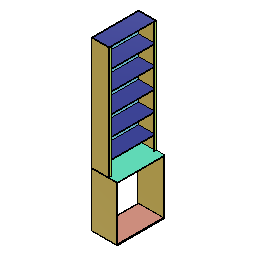
MS_BookShelves (Autodesk Fusion 360 design; units mm, degrees)
Autodesk Fusion 360 part; units mm, degrees
sketch "Part List" plane through (0, 0, 0) normal (1, 0, 0) x (0, 1, 0)
  line L0 (-117.4604, 5.2821) -> (-27.4764, 5.2821) construction
  line L1 (-27.4764, 5.2821) -> (-27.4764, 106.5384) construction
  line L2 (-27.4764, 106.5384) -> (-117.4604, 106.5384) construction
  line L3 (-117.4604, 106.5384) -> (-117.4604, 5.2821) construction
  dimension "d1" = 2
sketch "Room" plane through (0, 0, 0) normal (0, 0, 1) x (1, 0, 0)
  line L0 (922.3375, 3178.175) -> (2225.675, 3178.175) construction
  line L1 (0, 3178.175) -> (922.3375, 3178.175) construction
  line L2 (2225.675, 3178.175) -> (3114.675, 3178.175) construction
  line L3 (2259.0125, 0) -> (1363.6625, 0) construction
  line L4 (1363.6625, 46.449) -> (2259.0125, 46.449) construction
  line L5 (3114.675, 3178.175) -> (3630.6125, 3178.175) construction
  line L6 (0, 0) -> (0, 3178.175) construction
  line L7 (1363.6625, 0) -> (1363.6625, 46.449) construction
  line L8 (58.5758, 2317.75) -> (0, 2317.75) construction
  line L9 (0, 2403.475) -> (58.5758, 2403.475) construction
  line L10 (58.5758, 2403.475) -> (58.5758, 2317.75) construction
  line L11 (140.5097, 3178.175) -> (140.5097, 2420.9375) construction
  line L12 (0, 2317.75) -> (0, 2403.475) construction
  line L13 (0, 0) -> (3648.075, 0) construction
  line L14 (2259.0125, 46.449) -> (2259.0125, 0) construction
  point P0 (0, 2403.475)
  point P1 (0, 2317.75)
  point P2 (2259.0125, 0)
  point P3 (1363.6625, 0)
  dimension "d2" = 3648.075
  dimension "d3" = 895.35
  dimension "d4" = 1363.6625
  dimension "d5" = 1389.0625
  dimension "d6" = 3178.175
  dimension "d7" = 922.3375
  dimension "d8" = 1303.3375
  dimension "d9" = 889
  dimension "d10" = 515.9375
  dimension "d11" = 3630.6125
  dimension "d12" = 774.7
  dimension "d13" = 85.725
  dimension "d14" = 757.2375
  dimension "d15" = 90
  constraint coincident L6.start L13.start
  constraint horizontal L13
  constraint coincident P3 L13
  constraint coincident P2 L13
  constraint horizontal L3
  constraint vertical L7
  constraint horizontal L4
  constraint vertical L14
  constraint coincident P2 L3.start
  constraint perpendicular L6 L13
  constraint perpendicular L1 L6
  constraint parallel L0 L1
  constraint parallel L0 L2
  constraint parallel L2 L5
  constraint coincident P0 L6
  constraint coincident P1 L6
  constraint horizontal L9
  constraint vertical L10
  constraint horizontal L8
  constraint vertical L12
  constraint coincident P0 L9.start
  constraint coincident L11.start L1
  constraint perpendicular L1 L11
  measures "d2" distance of L13.end L6.start
  measures "d3" distance of P2 P3
  measures "d4" distance of L6.start P3
  measures "d5" distance of L13.end P2
  measures "d6" distance of L6.start L1.start
  measures "d7" distance of L1.start L0.start
  measures "d8" distance of L0.start L0.end
  measures "d9" distance of L0.end L2.end
  measures "d10" distance of L2.end L5.end
  measures "d11" distance of L1.start L5.end
  measures "d12" distance of L1.start P0
  measures "d13" distance of P0 P1
  measures "d14" distance of L11.start L11.end
  measures "d15" angle of L1 L11
sketch "Celing" plane through (0, 0, 0) normal (0, 0, 1) x (1, 0, 0)
  line L0 (0, 0, 2743.2) -> (3648.075, 0, 2743.2)
  line L1 (3648.075, 0, 2743.2) -> (3648.075, 3178.175, 2743.2)
  line L2 (3648.075, 3178.175, 2743.2) -> (0, 3178.175, 2743.2)
  line L3 (0, 3178.175, 2743.2) -> (0, 0, 2743.2)
  dimension "height" = 2743.2
  dimension "width" = 3648.075
  dimension "length" = 3178.175
ref_plane "WorkPlane1" through (0, 0, 0) normal (0, 1, 0) x (0, 0, 1) in component ">>WSSi_Sides"
sketch "Sketch1" plane through (0, 0, 0) normal (0, 1, 0) x (1, 0, 0) in component ">>WSSi_Sides"
  line L0 (6.35, 0) -> (266.7, 0)
  line L1 (266.7, 0) -> (266.7, -1739.9)
  line L2 (266.7, -1739.9) -> (6.35, -1739.9)
  line L3 (6.35, -1739.9) -> (6.35, 0)
  point P0 (6.35, 0)
  dimension "WSSi_Sides_YOrig" = 0
  dimension "WSSi_Sides_XOrig" = 6.35
  dimension "WSSi_Sides_Width" = 260.35
  dimension "WSSi_Sides_Length" = 1739.9
  constraint horizontal L0
  constraint vertical L1
  constraint horizontal L2
  constraint vertical L3
  constraint coincident P0 L0.start
  measures "WSSi_Sides_YOrig" vertical distance of origin L0.start
  measures "WSSi_Sides_XOrig" horizontal distance of origin L0.start
  measures "WSSi_Sides_Width" distance of P0 L0.end
  measures "WSSi_Sides_Length" distance of P0 L2.end
extrude "Extrude1" add sketch "Sketch1" along normal blind 12.7 makes body 1 in component ">>WSSi_Sides"
pattern_linear "00000000-0000-0000-0000-000000000000" [suppressed] in component ">WS - Sides"
ref_plane "WorkPlane1" through (0, 0, 0) normal (1, 0, 0) x (0, 1, 0) in component ">WS - Back"
sketch "Sketch1 (2)" plane through (0, 0, 0) normal (1, 0, 0) x (0, 1, 0) in component ">WS - Back"
  line L0 (0, 0) -> (736.6, 0)
  line L1 (736.6, 0) -> (736.6, 1739.9)
  line L2 (736.6, 1739.9) -> (0, 1739.9)
  line L3 (0, 1739.9) -> (0, 0)
  line L4 (12.7, 0) -> (723.9, 0)
  line L5 (723.9, 0) -> (723.9, 1727.2)
  line L6 (723.9, 1727.2) -> (12.7, 1727.2)
  line L7 (12.7, 1727.2) -> (12.7, 0)
  point P0 (12.7, 0)
  dimension "WS_Back_Width" = 736.6
  dimension "WS_Back_Length" = 1739.9
  dimension "WS_Back_YOrig" = 0
  dimension "WS_Back_XOrig" = 0
  dimension "WS_Back_Rabbit_Width" = 12.7
  dimension "WS_Back_NoRabbitWidth" = 711.2
  dimension "WS_Back_NoRabbit_Length" = 1727.2
  constraint horizontal L0
  constraint vertical L1
  constraint horizontal L2
  constraint vertical L3
  constraint coincident L0 P0
  constraint horizontal L4
  constraint vertical L5
  constraint horizontal L6
  constraint vertical L7
  constraint coincident P0 L4.start
  measures "WS_Back_Width" distance of L0.start L0.end
  measures "WS_Back_Length" distance of L0.start L2.end
  measures "WS_Back_YOrig" vertical distance of L0.start L3.end
  measures "WS_Back_XOrig" horizontal distance of L0.start L3.end
  measures "WS_Back_Rabbit_Width" distance of L0.start L4.start
  measures "WS_Back_NoRabbitWidth" distance of P0 L4.end
  measures "WS_Back_NoRabbit_Length" distance of P0 L6.end
extrude "Extrude1'" add sketch "Sketch1 (2)" along normal blind 12.7 separate body contours L0 L4 L5 L6 L7 makes body 2 in component ">WS - Back"
extrude "Extrude2" add sketch "Sketch1 (2)" along normal blind 6.35 contours L0 L1 L2 L3 L5 L6 L7 bodies 2 in component ">WS - Back"
ref_plane "WorkPlane1" through (12.7, 0, 0) normal (1, 0, 0) x (0, 1, 0) in component ">>WSS_Shelves"
sketch "Sketch1 (3)" plane through (12.7, 0, 0) normal (1, 0, 0) x (0, 1, 0) in component ">>WSS_Shelves"
  line L0 (12.7, 1727.2) -> (723.9, 1727.2)
  line L1 (723.9, 1727.2) -> (723.9, 1739.9)
  line L2 (723.9, 1739.9) -> (12.7, 1739.9)
  line L3 (12.7, 1739.9) -> (12.7, 1727.2)
  point P0 (12.7, 1727.2)
  dimension "WSS_Shelves_YOrig" = 1727.2
  dimension "WSS_Shelves_XOrig" = 12.7
  dimension "WSS_Shelves_Length" = 711.2
  dimension "WSS_Shelves_Thickness" = 12.7
  constraint horizontal L0
  constraint vertical L1
  constraint horizontal L2
  constraint vertical L3
  constraint coincident P0 L0.start
  measures "WSS_Shelves_YOrig" vertical distance of origin L0.start
  measures "WSS_Shelves_XOrig" horizontal distance of origin L0.start
  measures "WSS_Shelves_Length" distance of P0 L0.end
  measures "WSS_Shelves_Thickness" distance of P0 L2.end
extrude "Extrude1''" add sketch "Sketch1 (3)" along normal blind 254 separate body makes body 3 in component ">>WSS_Shelves"
pattern_linear "00000000-0000-0000-0000-000000000000'" [suppressed] in component ">WS - Shelves"
ref_plane "WorkPlane1" through (266.7, 0, 0) normal (1, 0, 0) x (0, 1, 0) in component ">WS - Molding"
sketch "Sketch1 (4)" plane through (266.7, 0, 0) normal (1, 0, 0) x (0, 1, 0) in component "WSM_Molding"
  line L0 (0, 0) -> (38.1, 0)
  line L1 (38.1, 0) -> (38.1, 1739.9)
  line L2 (38.1, 1739.9) -> (0, 1739.9)
  line L3 (0, 1739.9) -> (0, 0)
  dimension "WSM_Molding_OrigX" = 0
  dimension "WSM_Molding_OrigY" = 0
  dimension "WSM_Molding_Width" = 38.1
  dimension "WSM_Molding_Length" = 1739.9
  constraint horizontal L0
  constraint vertical L1
  constraint horizontal L2
  constraint vertical L3
  constraint coincident L0.start L3.end
  measures "WSM_Molding_OrigX" horizontal distance of L0.start L3.end
  measures "WSM_Molding_OrigY" vertical distance of L0.start L3.end
  measures "WSM_Molding_Width" distance of L0.start L0.end
  measures "WSM_Molding_Length" distance of L0.start L2.end
extrude "Extrude1'''" add sketch "Sketch1 (4)" along normal blind 12.7 separate body makes body 4 in component "WSM_Molding"
pattern_linear "00000000-0000-0000-0000-000000000000''" [suppressed] in component ">WS - Molding"
ref_plane "WorkPlane1" through (0, 0, -12.7) normal (0, 0, 1) x (1, 0, 0) in component ">>WCT_TableTop"
sketch "Sketch1 (5)" plane through (0, 0, -12.7) normal (0, 0, 1) x (1, 0, 0) in component ">>WCT_TableTop"
  line L0 (0, 0) -> (406.4, 0)
  line L1 (406.4, 0) -> (406.4, 736.6)
  line L2 (406.4, 736.6) -> (0, 736.6)
  line L3 (0, 736.6) -> (0, 0)
  dimension "WC_TableTop_OrigY" = 0
  dimension "WC_TableTop_OrigX" = 0
  dimension "WCT_TableTop_Width" = 406.4
  dimension "WCT_TableTop_Length" = 736.6
  constraint horizontal L0
  constraint vertical L1
  constraint horizontal L2
  constraint vertical L3
  constraint coincident L0.start L3.end
  measures "WC_TableTop_OrigY" horizontal distance of L0.start L3.end
  measures "WC_TableTop_OrigX" vertical distance of L0.start L3.end
  measures "WCT_TableTop_Width" distance of L0.start L0.end
  measures "WCT_TableTop_Length" distance of L0.start L2.end
extrude "Extrude1''''" add sketch "Sketch1 (5)" along normal blind 12.7 separate body makes body 5 in component ">>WCT_TableTop"
ref_plane "WorkPlane1" through (0, 0, -850.9) normal (0, 0, 1) x (1, 0, 0) in component ">>WCB_Bottom"
sketch "Sketch1 (6)" plane through (0, 0, -850.9) normal (0, 0, 1) x (1, 0, 0) in component ">>WCB_Bottom"
  line L0 (0, 0) -> (406.4, 0)
  line L1 (406.4, 0) -> (406.4, 736.6)
  line L2 (406.4, 736.6) -> (0, 736.6)
  line L3 (0, 736.6) -> (0, 0)
  line L4 (393.7, 12.7) -> (393.7, 723.9)
  line L5 (393.7, 723.9) -> (12.7, 723.9)
  line L6 (12.7, 723.9) -> (12.7, 12.7)
  line L7 (12.7, 12.7) -> (393.7, 12.7)
  dimension "WC_Bottom_OrigY" = 0
  dimension "WC_Bottom_OrigX" = 0
  dimension "WCB_Bottom_Width" = 406.4
  dimension "WCB_Bottom_Length" = 736.6
  constraint horizontal L0
  constraint vertical L1
  constraint horizontal L2
  constraint vertical L3
  constraint coincident L0.start L3.end
  measures "WC_Bottom_OrigY" vertical distance of L0.start L3.end
  measures "WC_Bottom_OrigX" horizontal distance of L0.start L3.end
  measures "WCB_Bottom_Width" distance of L0.start L0.end
  measures "WCB_Bottom_Length" distance of L0.start L2.end
extrude "Extrude1'''''" add sketch "Sketch1 (6)" along normal blind 12.7 separate body contours L4 L5 L6 L7 makes body 6 in component ">>WCB_Bottom"
extrude "Extrude2'" add sketch "Sketch1 (6)" along normal blind 6.35 bodies 6 in component ">>WCB_Bottom"
ref_plane "WorkPlane1" through (0, 0, 0) normal (0, 1, 0) x (0, 0, 1) in component ">>WCS_Sides"
sketch "Sketch1 (7)" plane through (0, 0, 0) normal (0, 1, 0) x (1, 0, 0) in component ">>WCS_Sides"
  line L0 (0, 844.55) -> (393.7, 844.55)
  line L1 (393.7, 844.55) -> (393.7, 12.7)
  line L2 (393.7, 12.7) -> (0, 12.7)
  line L3 (0, 12.7) -> (0, 844.55)
  point P0 (0, 844.55)
  dimension "WC_Sides_OrigX" = 0
  dimension "WCS_Sides_Width" = 393.7
  dimension "WCS_Sides_Length" = 831.85
  constraint horizontal L0
  constraint vertical L1
  constraint horizontal L2
  constraint vertical L3
  constraint coincident P0 L0.start
  measures "WC_Sides_OrigX" horizontal distance of origin L0.start
  measures "WCS_Sides_Width" distance of P0 L0.end
  measures "WCS_Sides_Length" distance of P0 L2.end
extrude "Extrude1''''''" add sketch "Sketch1 (7)" along normal blind 12.7 separate body makes body 7 in component ">>WCS_Sides"
pattern_linear "00000000-0000-0000-0000-000000000000'''" [suppressed] in component ">WC - Sides"
component "West Shelves" placed x (1, 0, 0) y (0, 1, 0) z (0, 0, 1) at (0, 0, 0)
component "West Cabinet" placed x (1, 0, 0) y (0, 1, 0) z (0, 0, 1) at (0, 0, 0)
component "West Toe Guard" placed x (1, 0, 0) y (0, 1, 0) z (0, 0, 1) at (0, 0, 0)
component "North Shelves" placed x (1, 0, 0) y (0, 1, 0) z (0, 0, 1) at (0, 0, 0)
component "North Cabinet" placed x (1, 0, 0) y (0, 1, 0) z (0, 0, 1) at (0, 0, 0)
component "North Toe Guard" placed x (1, 0, 0) y (0, 1, 0) z (0, 0, 1) at (0, 0, 0)
component ">WS - Sides" placed x (1, 0, 0) y (0, 1, 0) z (0, 0, 1) at (0, 0, 0) in component "West Shelves"
component ">WS - Back" placed x (1, 0, 0) y (0, 1, 0) z (0, 0, 1) at (0, 0, 0) in component "West Shelves"
component ">WS - Molding" placed x (1, 0, 0) y (0, 1, 0) z (0, 0, 1) at (0, 0, 0) in component "West Shelves"
component ">WS - Shelves" placed x (1, 0, 0) y (0, 1, 0) z (0, 0, 1) at (0, 0, 0) in component "West Shelves"
component "~~WC - Table Top" placed x (1, 0, 0) y (0, 1, 0) z (0, 0, 1) at (0, 0, 0) in component "West Cabinet"
component ">WC - Bottom" placed x (1, 0, 0) y (0, 1, 0) z (0, 0, 1) at (0, 0, 0) in component "West Cabinet"
component ">WC - Sides" placed x (1, 0, 0) y (0, 1, 0) z (0, 0, 1) at (0, 0, 0) in component "West Cabinet"
component ">WC - Back" placed x (1, 0, 0) y (0, 1, 0) z (0, 0, 1) at (0, 0, 0) in component "West Cabinet"
component ">WC - Front" placed x (1, 0, 0) y (0, 1, 0) z (0, 0, 1) at (0, 0, 0) in component "West Cabinet"
component ">WC - Doors" placed x (1, 0, 0) y (0, 1, 0) z (0, 0, 1) at (0, 0, 0) in component "West Cabinet"
component ">WC - Molding" placed x (1, 0, 0) y (0, 1, 0) z (0, 0, 1) at (0, 0, 0) in component "West Cabinet"
component ">WC - Shelves" placed x (1, 0, 0) y (0, 1, 0) z (0, 0, 1) at (0, 0, 0) in component "West Cabinet"
component "WTG - Front/Back" placed x (1, 0, 0) y (0, 1, 0) z (0, 0, 1) at (0, 0, 0) in component "West Toe Guard"
component "WTG - Left/Right" placed x (1, 0, 0) y (0, 1, 0) z (0, 0, 1) at (0, 0, 0) in component "West Toe Guard"
component "WTG - Brace" placed x (1, 0, 0) y (0, 1, 0) z (0, 0, 1) at (0, 0, 0) in component "West Toe Guard"
component ">>WSSi_Sides" placed x (1, 0, 0) y (0, 1, 0) z (0, 0, 1) at (0, 0, 0) in component ">WS - Sides"
component ">>WSSi_Sides" placed x (1, 0, 0) y (0, 1, 0) z (0, 0, 1) at (0, 723.9, 0) in component ">WS - Sides"
component "WSM_Molding" placed x (1, 0, 0) y (0, 1, 0) z (0, 0, 1) at (0, 0, 0) in component ">WS - Molding"
component "WSM_Molding" placed x (1, 0, 0) y (0, 1, 0) z (0, 0, 1) at (0, 698.5, 0) in component ">WS - Molding"
component ">>WCT_TableTop" placed x (1, 0, 0) y (0, 1, 0) z (0, 0, 1) at (0, 0, 0) in component "~~WC - Table Top"
component ">>WCB_Bottom" placed x (1, 0, 0) y (0, 1, 0) z (0, 0, 1) at (0, 0, 0) in component ">WC - Bottom"
component ">>WCS_Sides" placed x (1, 0, 0) y (0, 1, 0) z (0, 0, 1) at (0, 0, 0) in component ">WC - Sides"
component ">>WCS_Sides" placed x (1, 0, 0) y (0, 1, 0) z (0, 0, 1) at (0, 723.9, 0) in component ">WC - Sides"
component "WC_F - Top/Bottom" placed x (1, 0, 0) y (0, 1, 0) z (0, 0, 1) at (0, 0, 0) in component ">WC - Front"
component "WC_F - Left/Right" placed x (1, 0, 0) y (0, 1, 0) z (0, 0, 1) at (0, 0, 0) in component ">WC - Front"
component "WC_D - Top/Bottom" placed x (1, 0, 0) y (0, 1, 0) z (0, 0, 1) at (0, 0, 0) in component ">WC - Doors"
component "WC_D - Left/Right" placed x (1, 0, 0) y (0, 1, 0) z (0, 0, 1) at (0, 0, 0) in component ">WC - Doors"
component "WC_D - Center" placed x (1, 0, 0) y (0, 1, 0) z (0, 0, 1) at (0, 0, 0) in component ">WC - Doors"
component "WC_M - West Top/Bottom" placed x (1, 0, 0) y (0, 1, 0) z (0, 0, 1) at (0, 0, 0) in component ">WC - Molding"
component "WC_M - West Left/Right" placed x (1, 0, 0) y (0, 1, 0) z (0, 0, 1) at (0, 0, 0) in component ">WC - Molding"
component "WC_M - North Top/Bottom" placed x (1, 0, 0) y (0, 1, 0) z (0, 0, 1) at (0, 0, 0) in component ">WC - Molding"
component "WC_M - North Left/Right" placed x (1, 0, 0) y (0, 1, 0) z (0, 0, 1) at (0, 0, 0) in component ">WC - Molding"
component ">>WSS_Shelves" placed x (1, 0, 0) y (0, 1, 0) z (0, 0, 1) at (0, 0, 0) in component ">WS - Shelves"
component ">>WSS_Shelves" placed x (1, 0, 0) y (0, 1, 0) z (0, 0, 1) at (0, 0, -304.8) in component ">WS - Shelves"
component ">>WSS_Shelves" placed x (1, 0, 0) y (0, 1, 0) z (0, 0, 1) at (0, 0, -609.6) in component ">WS - Shelves"
component ">>WSS_Shelves" placed x (1, 0, 0) y (0, 1, 0) z (0, 0, 1) at (0, 0, -914.4) in component ">WS - Shelves"
component ">>WSS_Shelves" placed x (1, 0, 0) y (0, 1, 0) z (0, 0, 1) at (0, 0, -1219.2) in component ">WS - Shelves"
component ">>WSS_Shelves" placed x (1, 0, 0) y (0, 1, 0) z (0, 0, 1) at (0, 0, -1524) in component ">WS - Shelves"
equation "room_W_wall = 10'-0\" + 5\" + 0.125 in"
equation "room_distance_to_ceiling = 9 ft"
equation "room_shelves_depth = 11\" + 0'- 1/16\""
equation "room_shelves_width = 5'-0\" + 0'- 9/16\""
equation "room_shelves_height = 58.75 in"
equation "room_doors_left = 2'-0\" + 5\" + 0'- 13/16\""
equation "room_doors_right = room_doors_left"
equation "room_doorframe_left = 2'-0\" + 11\""
equation "room_doorframe_right = room_doorframe_left"
equation "room_NS_wall = 11'-0\" + 10.75 in"
equation "room_S_wall_right = 4'-0\" + 5\" + 0'- 11/16\""
equation "room_S_wall_left = 4'-0\" + 6\" + 0'- 11/16\""
equation "room_S_wall_window = 2'-0\" + 11.25 in"
equation "room_S_wall_total = room_S_wall_left + room_S_wall_right + room_S_wall_window"
equation "room_N_wall_p1 = 3'-0\" + 0'- 5/16\""
equation "room_N_wall_p2 = 4'-0\" + 3\" + 0'- 5/16\""
equation "room_N_wall_p3 = 1'-0\" + 8\" + 0'- 5/16\""
equation "room_W_outlet_NWallToRight = 2'-0\" + 6.5 in"
equation "room_W_outlet_floorToBtm = 11\" + 0'- 5/8\""
equation "room_W_outlet_floorToTop = 1'-0\" + 4\" + 0'- 11/16\""
equation "room_W_outlet_NWallToLeft = 2'-0\" + 9\" + 0'- 7/8\""
equation "room_W_outlet_length = room_W_outlet_floorToTop - room_W_outlet_floorToBtm"
equation "room_W_outlet_width = room_W_outlet_NWallToLeft - room_W_outlet_NWallToRight"
equation "material_thickness = 0.5 in"
equation "Shared_WSS_Shelves_Width = 10 in"
equation "Shared_WestCabinet_TotalHeight = 3'-0\" - cabinet_toe_guard"
equation "Shared_W_Total_Width = room_W_wall - 36\""
equation "Shared_W_Cabinet_Depth = Shared_WSS_Shelves_Width + 6\""
equation "shlf_S_ttl_width = room_S_wall_right - Shared_W_Cabinet_Depth - 1 in"
equation "Shared_W_Total_Height = room_distance_to_ceiling - Shared_WestCabinet_TotalHeight - material_thickness - cabinet_toe_guard - 3\""
equation "cabinet_toe_guard = material_toe_width"
equation "Shared_W_NumOfSections = 3"
equation "Shared_WSS_Shelves_Length = Shared_W_Section_Width - ( Shared_WCS_Sides_Thickness * 2 )"
equation "shlf_W_distanceBTWShelves = 12 in"
equation "shlf_W_numOfShelves = floor(Shared_W_Total_Height / shlf_W_distanceBTWShelves) + 1"
equation "toe_W_length = Shared_W_Section_Width"
equation "toe_W_width = Shared_W_Cabinet_Depth - cabinet_toe_guard"
equation "material_toe_width = 3.0 in"
equation "material_toe_thickness = 1.5 in"
equation "toe_bracket = 6 in"
equation "cabinet_W_tblTopLength = ( Shared_WSS_Shelves_Length + ( material_thickness * 2 ) ) * 3"
equation "cabinet_W_side_width = Shared_W_Cabinet_Depth - ( material_thickness * 2 )"
equation "cabinet_W_side_length = Shared_WestCabinet_TotalHeight - ( material_thickness / 2 )"
equation "cabinet_W_back_length = Shared_WestCabinet_TotalHeight - ( material_thickness / 2 )"
equation "cabinet_W_back_width = toe_W_length"
equation "cabinet_W_btm_length = toe_W_length"
equation "cabinet_W_front_TB_length = cabinet_W_btm_length"
equation "cabinet_W_front_width = cabinet_bezzle"
equation "cabinet_W_front_LR_length = cabinet_W_side_length - ( cabinet_W_front_width * 2 )"
equation "cabinet_bezzle = 3 in"
equation "Shared_WSSi_Sides_length = Shared_W_Total_Height"
equation "cabinet_W_door_offset = ( cabinet_bezzle / 2 ) + 0.25 in"
equation "cabinet_W_door_TB_length = ( cabinet_W_front_TB_length / 2 ) - cabinet_W_door_offset - ( cabinet_W_doors_spaceBTWDoors / 2 )"
equation "cabinet_W_door_TB_width = cabinet_door_bezzle"
equation "cabinet_W_doors_spaceBTWDoors = 0.25 in"
equation "cabinet_W_door_LR_length = cabinet_W_side_length - ( cabinet_W_door_offset * 2 ) - ( cabinet_W_door_TB_width * 2 )"
equation "cabinet_door_bezzle = 2 in"
equation "cabinet_W_door_LR_width = cabinet_door_bezzle"
equation "cabinet_W_door_rabbit = material_door_center"
equation "cabinet_W_door_center_width = cabinet_W_door_TB_length - ( cabinet_W_door_LR_width * 2 ) + ( cabinet_W_door_rabbit )"
equation "cabinet_W_door_center_length = cabinet_W_door_LR_length + cabinet_W_door_rabbit"
equation "cabinet_W_door_center_thickness = material_door_center"
equation "material_door_center = 0.25 in"
equation "cabinet_W_trim_W_length = cabinet_W_tblTopLength + material_thickness" comment "material thickness is to accomidate for champher"
equation "cabinet_W_trim_W_width = material_thickness + cabinet_W_door_offset - 0.25 in"
equation "cabinet_W_trim_N_length = Shared_W_Cabinet_Depth + material_thickness"
equation "cabinet_W_trim_N_width = cabinet_W_trim_W_width" comment "b/c it needs to match the other trim"
equation "shlf_W_molding_width = 1.5 in"
equation "shlf_W_molding_length = Shared_WSSi_Sides_length"
equation "shlf_W_molding_origin = 0.001 in"
equation "cabinet_W_trim_W_LR_length = ( cabinet_W_front_width * 2 ) + cabinet_W_front_LR_length - ( cabinet_W_trim_W_LR_width * 2 )"
equation "cabinet_W_trim_W_LR_width = shlf_W_molding_width"
equation "height = room_distance_to_ceiling"
equation "width = room_S_wall_total"
equation "length = room_W_wall"
equation "WSSi_Sides_ZOrig = 0 ft"
equation "WSSi_Sides_XOrig = Shared_WS_Back_Rabbit_Depth"
equation "WSSi_Sides_Width = Shared_WSSi_Sides_Width"
equation "WSSi_Sides_Length = Shared_WSSi_Sides_length"
equation "shlf_W_shlf_thickness = material_thickness"
equation "WSSi_Sides_Thickness = Shared_WSSi_Sides_Thickness"
equation "WS_Sides_NumOfSides = 2"
equation "WS_Sides_DistanceBTWSides = Shared_WS_Sides_DistanceBTWSides"
equation "WS_Back_ZOrig = 0 in"
equation "WS_Back_Width = Shared_WS_Back_Width"
equation "WS_Back_Length = Shared_W_Total_Height"
equation "WS_Back_Thickness = Shared_WS_Back_Thickness"
equation "WS_Back_Rabbit_Depth = Shared_WS_Back_Rabbit_Depth"
equation "Shared_WS_Back_Thickness = material_thickness"
equation "WS_Back_Rabbit_Width = Shared_WSSi_Sides_Thickness"
equation "WS_Back_NoRabbitWidth = WS_Back_Width - ( Shared_WSS_Shelves_Thickness * 2 )"
equation "WS_Back_NoRabbit_Length = WS_Back_Length - Shared_WSS_Shelves_Thickness"
equation "WSS_Shelves_ZOrig = Shared_WS_Back_Thickness"
equation "WSS_Shelves_YOrig = Shared_WSSi_Sides_length - Shared_WSS_Shelves_Thickness"
equation "WSS_Shelves_XOrig = Shared_WSSi_Sides_Thickness"
equation "WSS_Shelves_Length = Shared_WSS_Shelves_Length"
equation "WSS_Shelves_Thickness = Shared_WSS_Shelves_Thickness"
equation "WSS_Shelves_Width = Shared_WSS_Shelves_Width"
equation "Shared_WS_Sides_DistanceBTWSides = -( Shared_W_Section_Width - Shared_WSSi_Sides_Thickness )"
equation "Shared_WSS_Shelves_Thickness = 0.5 in"
equation "Shared_WSSi_Sides_Thickness = material_thickness"
equation "WS_Shelves_NumOfShelves = shlf_W_numOfShelves"
equation "WS_Shelves_DistBTWShelves = -( shlf_W_distanceBTWShelves )"
equation "Shared_WS_Back_Rabbit_Depth = Shared_WS_Back_Thickness / 2"
equation "WS_Molding_OrigZ = Shared_WS_Back_Rabbit_Depth + Shared_WSSi_Sides_Width"
equation "WSM_Molding_Length = Shared_WSSi_Sides_length"
equation "WSM_Molding_Thickness = Shared_WSM_Molding_Thickness"
equation "Shared_WSM_Molding_Thickness = material_thickness"
equation "Shared_WSSi_Sides_Width = Shared_WSS_Shelves_Width + Shared_WS_Back_Rabbit_Depth"
equation "WSM_Molding_Num = 2"
equation "WSM_Molding_SpaceBTWMolding = Shared_WS_Back_Width - WSM_Molding_Width"
equation "Shared_WS_Back_Width = Shared_WSS_Shelves_Length + ( Shared_WSSi_Sides_Thickness * 2 )"
equation "WC_TableTop_OrigZ = -( Shared_WCT_TableTop_Thickness )"
equation "WCT_TableTop_Width = Shared_W_Cabinet_Depth"
equation "WCT_TableTop_Length = Shared_WS_Back_Width"
equation "WCT_TableTop_Thickness = Shared_WCT_TableTop_Thickness"
equation "Shared_WCT_TableTop_Thickness = material_thickness"
equation "WC_Bottom_OrigZ = -( abs(WC_Sides_OrigZ) + WCB_Bottom_Rabbit_Depth )"
equation "WCB_Bottom_Width = Shared_W_Cabinet_Depth"
equation "WCB_Bottom_Length = Shared_WSS_Shelves_Length + ( Shared_WCS_Sides_Thickness * 2 )"
equation "WCB_Bottom_Rabbit_Width = -( Shared_WCB_Bottom_Thickness )"
equation "WCB_Bottom_Thickness = Shared_WCB_Bottom_Thickness"
equation "WCB_Bottom_Rabbit_Depth = Shared_WCB_Bottom_Thickness / 2"
equation "Shared_WCB_Bottom_Thickness = material_thickness"
equation "WC_Sides_OrigY = 0 in"
equation "WC_Sides_OrigZ = -( WCS_Sides_Length + Shared_WCT_TableTop_Thickness )"
equation "WCS_Sides_Width = Shared_W_Cabinet_Depth - abs(WCB_Bottom_Rabbit_Width)"
equation "WCS_Sides_Length = Shared_WestCabinet_TotalHeight - WCB_Bottom_Rabbit_Depth"
equation "WCS_Sides_Thickness = Shared_WCS_Sides_Thickness"
equation "Shared_WCS_Sides_Thickness = material_thickness"
equation "Shared_W_Section_Width = floor(Shared_W_Total_Width / Shared_W_NumOfSections)"
equation "WC_Sides_NumOfSides = 2"
equation "WC_Sides_DistBTWSides = -( Shared_W_Section_Width - WCS_Sides_Thickness )"
